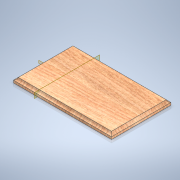
# Autodesk Inventor part: Base
Saved by Autodesk Inventor 2020.2 (Build 242310000, 310)
## iProperties
Created: 2020-02-25
Part Number: Base
Material: Wood (Birch)
Document SubType Name: Modeling
Designer: sdekr
Density: 0.55 g/cm^3
Appearance: Birch - Natural Polished
Author: sdekr
Autodesk Inventor part; units mm, degrees
ref_plane "YZ Plane" through (0, 0, 0) normal (1, 0, 0) x (0, 1, 0)
ref_plane "XZ Plane" through (0, 0, 0) normal (0, 1, 0) x (-1, 0, 0)
ref_plane "XY Plane" through (0, 0, 0) normal (0, 0, 1) x (1, 0, 0)
sketch "Sketch1" plane through (0, 0, 0) normal (0, 1, 0) x (-1, 0, 0)
  line L0 (0, 0) -> (330, 0)
  line L1 (330, 0) -> (330, -200)
  line L2 (330, -200) -> (0, -200)
  line L3 (0, -200) -> (0, 0)
  dimension "d0" = 330
  dimension "d1" = 200
  constraints: 8 end point, 2 parallel, 1 horizontal, 1 perpendicular
  measures "d0" distance of L1.end L2.end
  measures "d1" distance of L0.end L1.end
extrude "Extrusion1" add sketch "Sketch1" along normal blind 16
ref_plane "Work Plane1" through (-330, 0, -100) normal (0, 0, 1) x (1, 0, 0)
ref_plane "Work Plane2" through (-250, 0, -200) normal (-1, 0, 0) x (0, 0, 1)
fillet "Fillet3" radius 8 4 edges at (-165, 16, 0) (-330, 16, -100) (-165, 16, -200) (0, 16, -100) inverted yes
body "Solid1"
